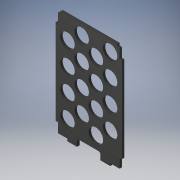
# Autodesk Inventor part: EBF_001.1-top-plate_cup-holder
Saved by Autodesk Inventor 2019 (Build 230136000, 136)
## iProperties
Created: 2019-02-28
Part Number: EBF_001.1-top-plate_cup-holder
Material: Generic
Document SubType Name: Modeling
Designer: Rene
Density: 1 g/cm^3
Appearance: Smooth - Black
Author: Rene
Autodesk Inventor part; units mm, degrees
ref_plane "YZ Plane" through (0, 0, 0) normal (1, 0, 0) x (0, 1, 0)
ref_plane "XZ Plane" through (0, 0, 0) normal (0, 1, 0) x (-1, 0, 0)
ref_plane "XY Plane" through (0, 0, 0) normal (0, 0, 1) x (1, 0, 0)
sketch "Sketch1" plane through (0, 0, 0) normal (0, 0, 1) x (1, 0, 0)
  line L0 (-70, -115) -> (70, -115)
  line L1 (70, -115) -> (70, 115)
  line L2 (70, 115) -> (-70, 115)
  line L3 (-70, 115) -> (-70, -115)
  point P0 (0, 0)
  dimension "width" = 140
  dimension "d1" = 70
  dimension "d2" = 230
  dimension "d3" = 115
  constraints: 8 end point, 2 parallel, 1 horizontal, 1 perpendicular
  measures "width" distance of L0.start L0.end
  measures "d1" horizontal distance of point (0, 0) L0.start
  measures "d2" distance of L2.end L0.start
  measures "d3" vertical distance of point (0, 0) L0.start
extrude "Extrusion1" add sketch "Sketch1" along normal blind 5
sketch "Sketch2" plane through (0, 0, 5) normal (0, 0, 1) x (1, 0, 0)
  circle A0 centre (-45, 69) radius 15.5
  circle A1 centre (-15, 93) radius 15.5
  point P0 (0, 0)
  dimension "d6" = 31
  dimension "d7" = 69
  dimension "d8" = 45
  dimension "d17" = 31
  dimension "d18" = 30
  dimension "d19" = 24
  constraints: 2 centre point
  measures "d6" diameter of A0
  measures "d7" vertical distance of A0.centre point (0, 0)
  measures "d8" horizontal distance of A0.centre point (0, 0)
  measures "d17" diameter of A1
  measures "d18" horizontal distance of A1.centre A0.centre
  measures "d19" vertical distance of A1.centre A0.centre
extrude "Extrusion2" cut sketch "Sketch2" against normal blind 5
pattern_linear "Rectangular Pattern2" count 2 spacing 60 along (1, 0, 0) count 4 spacing 48 along (0, -1, 0) of "Extrusion2"
sketch "Sketch3" plane through (0, 0, 5) normal (0, 0, 1) x (1, 0, 0)
  line L0 (-70, -115) -> (70, -115) projected
  line L1 (-70, -115) -> (-45, -115)
  line L2 (-45, -115) -> (-45, -110)
  line L3 (-45, -110) -> (-70, -110)
  line L4 (-70, -110) -> (-70, -115)
  line L5 (-70, 115) -> (-70, -115) projected
  line L6 (-70, 115) -> (-60, 115)
  line L7 (-60, 115) -> (-60, 110)
  line L8 (-60, 110) -> (-70, 110)
  line L9 (-70, 110) -> (-70, 115)
  line L10 (-70, -115) -> (-65, -115)
  line L11 (-65, -115) -> (-65, -90)
  line L12 (-65, -90) -> (-70, -90)
  line L13 (-70, -90) -> (-70, -115)
  line L14 (-70, 115) -> (-65, 115)
  line L15 (-65, 115) -> (-65, 90)
  line L16 (-65, 90) -> (-70, 90)
  line L17 (-70, 90) -> (-70, 115)
  point P0 (0, 0)
  dimension "d26" = 5
  dimension "d27" = 25
  dimension "d28" = 5
  dimension "d29" = 10
  dimension "d30" = 5
  dimension "d31" = 25
  dimension "d32" = 5
  dimension "d33" = 25
  constraints: 32 end point, 8 parallel, 4 horizontal, 4 perpendicular
  measures "d26" distance of L3.end L0.start
  measures "d27" distance of L2.end L3.end
  measures "d28" distance between parallel lines of L6 L8
  measures "d29" distance of L5.start L6.end
  measures "d30" distance of L11.end L12.end
  measures "d31" distance of L10.end L11.end
  measures "d32" distance of L15.end L16.end
  measures "d33" distance of L14.end L15.end
extrude "Extrusion3" cut sketch "Sketch3" against normal blind 10
mirror "Mirror1" about plane through (0, 0, 0) normal (1, 0, 0) of "Extrusion3"
sketch "Sketch4" plane through (0, 0, 5) normal (0, 0, 1) x (1, 0, 0)
  line L0 (-45, -115) -> (45, -115) projected
  line L1 (-25, -115) -> (25, -115)
  line L2 (25, -115) -> (25, -100)
  line L3 (25, -100) -> (-25, -100)
  line L4 (-25, -100) -> (-25, -115)
  point P0 (0, 0)
  dimension "d36" = 25
  dimension "d37" = 50
  dimension "d38" = 15
  constraints: 8 end point, 2 parallel, 1 horizontal, 1 perpendicular, 1 point on line
  measures "d36" horizontal distance of point (0, 0) L1.start
  measures "d37" distance of L2.end L3.end
  measures "d38" distance of L3.end L1.start
extrude "Extrusion4" cut sketch "Sketch4" against normal blind 10
fillet "Fillet1" radius 5 2 edges at (-25, -100, 2.5) (25, -100, 2.5)
equation "\"d1\" = 0.5 * width"
equation "\"d3\" = 0.5 * d2"
equation "\"d17\" = d6"
equation "\"d22\" = 2 * d18"
equation "\"d25\" = 2 * d19"
equation "\"d30\" = d26"
equation "\"d31\" = d27"
equation "\"d32\" = d28"
equation "\"d36\" = 0.5 * d37"
body "Solid1"
